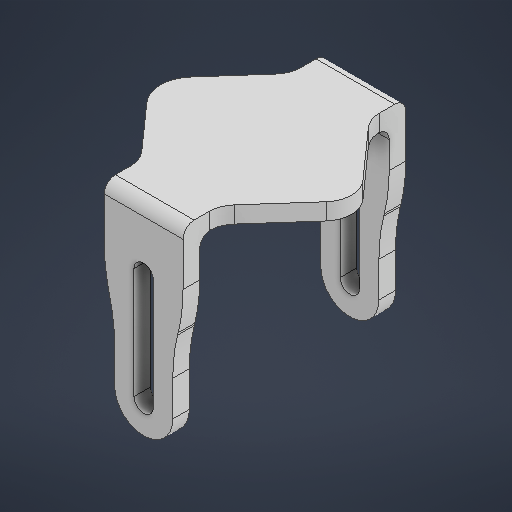
# Autodesk Inventor part: SoporteSensorDeInterrupcionesEJEX
Saved by Autodesk Inventor 2027 (Build 310192000, 192)
## iProperties
Created: 2026-05-01
Part Number: SoporteSensorDeInterrupcionesEJEX
Material: Generic
Document SubType Name: Modeling
Designer: 06aar
Density: 1 g/cm^3
Appearance: Default
Author: 06aar
Autodesk Inventor part; units mm, degrees
ref_plane "YZ Plane" through (0, 0, 0) normal (1, 0, 0) x (0, 1, 0)
ref_plane "XZ Plane" through (0, 0, 0) normal (0, 1, 0) x (-1, 0, 0)
ref_plane "XY Plane" through (0, 0, 0) normal (0, 0, 1) x (1, 0, 0)
sketch "Sketch1" plane through (0, 0, 0) normal (0, 1, 0) x (-1, 0, 0)
  line L0 (7.1, -20.1) -> (-7.1, -20.1)
  line L1 (-7.1, -20.1) -> (-7.1, 20.1)
  line L2 (-7.1, 20.1) -> (7.1, 20.1)
  line L3 (7.1, 20.1) -> (7.1, -20.1)
  line L4 (7.1, -20.1) -> (-7.1, 20.1) construction
  line L5 (-7.1, -20.1) -> (7.1, 20.1) construction
  circle A0 centre (0, 12.1) radius 2
  point P0 (0, 0)
  dimension "d0" = 14.2
  dimension "d1" = 40.2
  dimension "d4" = 4
  dimension "d5" = 8
  dimension "d6" = 7.1
  constraints: 12 end point, 2 midpoint, 2 parallel, 1 centre point, 1 horizontal, 1 perpendicular
  measures "d0" distance of L1.end L2.end
  measures "d1" distance of L2.end L0.start
  measures "d4" diameter of A0
  measures "d5" distance from line of L2 A0.centre
  measures "d6" distance from line of L3 A0.centre
extrude "Extrusion1" add sketch "Sketch1" along normal blind 3 contours L0 L1 L2 L3 | A0
sketch "Sketch2" plane through (-7.1, 0, 20.1) normal (0, 0, 1) x (1, 0, 0)
  line L0 (7.1, -28) -> (7.1, -8) construction
  line L1 (8.85, -28) -> (8.85, -8)
  line L2 (5.35, -8) -> (5.35, -28)
  arc A0 (5.35, -28) -> (8.85, -28) centre (7.1, -28) ccw
  arc A1 (8.85, -8) -> (5.35, -8) centre (7.1, -8) ccw
  line L3 (0, 0) -> (0, 3) projected
  line L4 (0, 0) -> (14.2, 0) projected
  line L5 (1.85, -28) -> (1.85, -8)
  arc A2 (12.35, -8) -> (1.85, -8) centre (7.1, -8) ccw
  line L6 (12.35, -8) -> (12.35, -28)
  arc A3 (1.85, -28) -> (12.35, -28) centre (7.1, -28) ccw
  line L7 (0, 0) -> (0, -10.5)
  line L8 (0, -10.5) -> (1.85, -18)
  line L9 (14.2, 0) -> (14.2, -10.5)
  line L10 (14.2, -10.5) -> (12.35, -18)
  point P0 (7.1, 0)
  point P1 (7.1, -18)
  point P2 (8.85, -18)
  dimension "d7" = 7.1
  dimension "d8" = 3.5
  dimension "d9" = 20
  dimension "d10" = 18
  dimension "d11" = 3.5
  constraints: 20 end point, 8 point on circle, 4 centre point, 4 midpoint, 4 tangent, 3 vertical, 2 parallel, 3 other
  measures "d7" distance between parallel lines of L3 L0
  measures "d8" distance from line of point (8.85, -18) L2
  measures "d9" distance of L0.start L0.end
  measures "d10" distance from line of L4 point (7.1, -18)
  measures "d11" distance between parallel lines of L5 L2
extrude "Extrusion2" add sketch "Sketch2" against normal blind 3
mirror "Mirror1" about plane through (0, 0, 0) normal (0, 0, 1) of "Extrusion2"
fillet "Fillet1" radius 30 8 edges at (7.1, -10.5, 18.6) (5.25, -18, 18.6) (-7.1, -10.5, 18.6) (-5.25, -18, 18.6) (7.1, -10.5, -18.6) (5.25, -18, -18.6) (-7.1, -10.5, -18.6) (-5.25, -18, -18.6)
sketch "Sketch3" plane through (0, 3, 0) normal (0, 1, 0) x (1, 0, 0)
  line L0 (-7.1, -13.5) -> (7.1, -13.5) projected
  line L1 (-7.1, -13.5) -> (-19.1, 0)
  line L2 (7.1, 13.5) -> (-7.1, 13.5) projected
  line L3 (-19.1, 0) -> (-7.1, 13.5)
  line L4 (-7.1, 13.5) -> (-7.1, -13.5)
  line L5 (-7.1, 20.1) -> (-7.1, -20.1) projected
  line L6 (-7.1, 0) -> (-19.1, 0)
  point P0 (0, 0)
  point P1 (-7.1, 0)
  point P2 (-7.1, 14.5)
  point P3 (-7.1, -14.5)
  dimension "d17" = 12
  constraints: 8 end point, 2 midpoint, 2 perpendicular
  measures "d17" distance of point (-7.1, 0) L1.end
extrude "Extrusion3" add sketch "Sketch3" against normal blind 3
fillet "Fillet4" radius 6 1 edges at (-19.1, 1.5, 0)
fillet "Fillet5" radius 5 2 edges at (-7.1, 1.5, 13.5) (-7.1, 1.5, -13.5)
mirror "Mirror2" about plane through (0, 0, 0) normal (1, 0, 0) of "Extrusion3"
fillet "Fillet6" radius 5 2 edges at (7.1, 1.5, 13.5) (7.1, 1.5, -13.5)
fillet "Fillet7" radius 5 1 edges at (19.1, 1.5, 0)
fillet "Fillet8" radius 2 4 edges at (0, 3, 20.1) (0, 3, -20.1) (0, 0, -17.1) (0, 0, 17.1)
body "Solid1"
